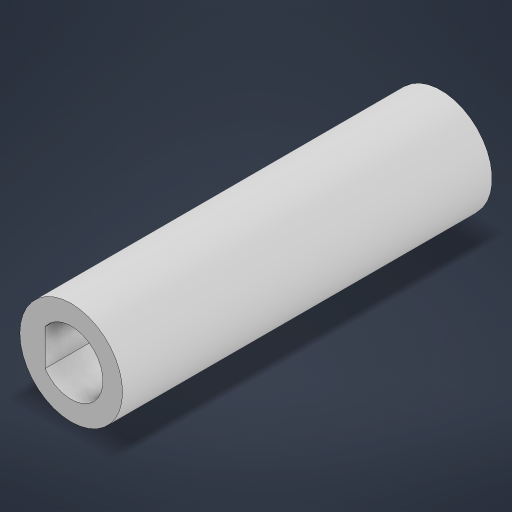
# Autodesk Inventor part: TestingWinch
Saved by Autodesk Inventor 2024 (Build 280153000, 153)
## iProperties
Created: 2024-03-11
Part Number: TestingWinch
Material: Generic
Document SubType Name: Modeling
Designer: avsar
Density: 1 g/cm^3
Appearance: Default
Author: avsar
Autodesk Inventor part; units mm, degrees
ref_plane "YZ Plane" through (0, 0, 0) normal (1, 0, 0) x (0, 1, 0)
ref_plane "XZ Plane" through (0, 0, 0) normal (0, 1, 0) x (-1, 0, 0)
ref_plane "XY Plane" through (0, 0, 0) normal (0, 0, 1) x (1, 0, 0)
sketch "Sketch1" plane through (0, 0, 0) normal (0, 0, 1) x (1, 0, 0)
  arc A0 (-4.5, -2.1795) -> (-4.5, 2.1795) centre (0, 0) ccw
  line L0 (-4.5, 2.1795) -> (-4.5, -2.1795)
  arc A1 (-4.5, 2.1795) -> (-4.5, -2.1795) centre (0, 0) ccw construction
  arc A2 (-4.6, -2.2023) -> (-4.6, 2.2023) centre (0, 0) ccw construction
  line L1 (-4.6, -2.2023) -> (-4.6, 2.2023) construction
  circle A3 centre (0, 0) radius 8 construction
  dimension "d0" = 10
  dimension "d1" = 4.359
  dimension "d2" = 0.1
  dimension "d3" = 16
  constraints: 6 point on circle, 4 centre point, 4 end point, 3 coincident, 1 vertical, 1 other
  measures "d0" diameter of A0
  measures "d1" distance of L0.start L0.end
  measures "d2" radial gap between concentric circles of A0 A2
  measures "d3" diameter of A3
extrude "Extrusion1" add sketch "Sketch1" along normal blind 24
sketch "Sketch3" plane through (0, 0, 24) normal (0, 0, 1) x (1, 0, 0)
  arc A0 (-2.4476, 1.7348) -> (-2.4476, -1.7348) centre (0, 0) ccw construction
  line L0 (0, 0) -> (-2.4476, -1.7348) construction
  line L1 (0, 0) -> (-2.4476, 1.7348) construction
  arc A1 (-2.4476, -1.7348) -> (-2.4476, 1.7348) centre (0, 0) ccw construction
  line L2 (-2.4476, 1.7348) -> (-2.4476, -1.7348) construction
  arc A2 (-2.5476, -1.7663) -> (-2.5476, 1.7663) centre (0, 0) ccw
  line L3 (-2.5476, -1.7663) -> (-2.5476, 1.7663)
  circle A3 centre (0, 0) radius 5
  point P0 (-4.5, 2.1795)
  dimension "d10" = 3
  dimension "d11" = 289.344
  dimension "d12" = 0.1
  constraints: 8 end point, 6 point on circle, 3 centre point, 3 coincident, 1 vertical, 4 other
  measures "d10" radius of A0
  measures "d12" radial gap between concentric circles of A1 A2
extrude "Extrusion3" add sketch "Sketch3" along normal blind 12
body "Solid1"
